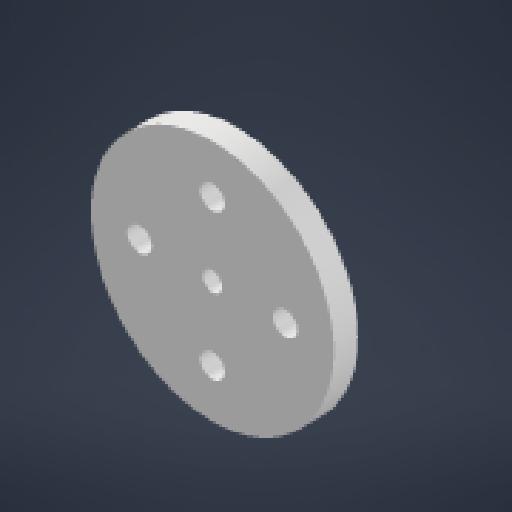
# Autodesk Inventor part: Part25
Saved by Autodesk Inventor 2027.1 (Build 311270010, 270A)
## iProperties
Created: 2026-09-29
Part Number: Part25
Material: Generic
Document SubType Name: Modeling
Designer: daniel
Density: 1 g/cm^3
Appearance: Default
Author: daniel
Autodesk Inventor part; units mm, degrees
ref_plane "YZ Plane" through (0, 0, 0) normal (1, 0, 0) x (0, 1, 0)
ref_plane "XZ Plane" through (0, 0, 0) normal (0, 1, 0) x (-1, 0, 0)
ref_plane "XY Plane" through (0, 0, 0) normal (0, 0, 1) x (1, 0, 0)
sketch "Sketch1" plane through (0, 0, 0) normal (0, 0, 1) x (1, 0, 0)
  circle A0 centre (0, 0) radius 2
  circle A1 centre (0, 0) radius 25
  circle A2 centre (0, 0) radius 3.5
  line L0 (-2, -2.8723) -> (-2, 2.8723)
  line L1 (-2.8723, 2) -> (2.8723, 2)
  line L2 (-2.8723, -2) -> (2.8723, -2)
  line L3 (2, -2.8723) -> (2, 2.8723)
  point P0 (2, -2)
  point P1 (2, 0)
  point P2 (-2, 0)
  point P3 (-2, -2)
  point P4 (2, 2)
  point P5 (-2, 2)
  dimension "d4" = 7
  dimension "d0" = 4
  dimension "d1" = 50
  constraints: 8 end point, 3 coincident, 2 centre point, 2 horizontal, 2 vertical, 10 other
  measures "d0" diameter of A0
  measures "d1" diameter of A1
extrude "Extrusion1" add sketch "Sketch1" along normal blind 5 contours L3 L2 A0 | L3 L1 A2 L2 | A0 L1 L3 | A0 L0 L1 | L1 L0 A2 L3 | L2 L0 A0 | L2 L3 A2 L0 | L2 A2 L3 | L3 A2 L1 | L0 L2 A2 L1 | L1 A2 L0 | L0 A2 L2 | A1
extrude "Extrusion2" add sketch "Sketch1" against normal blind 5 contours L3 L2 A0 | A0 L1 L3 | A0 L0 L1 | L1 L0 A2 L3 | L2 L0 A0 | L2 L3 A2 L0 | L2 A2 L3 | L3 A2 L1 | L1 A2 L0 | L0 A2 L2
sketch "Sketch2" plane through (0, 0, 5) normal (0, 0, 1) x (1, 0, 0)
  circle A0 centre (0, 0) radius 2 projected
  circle A1 centre (0, 0) radius 15
  circle A2 centre (-15, 0) radius 2.5
  circle A3 centre (0, 15) radius 2.5
  circle A4 centre (15, 0) radius 2.5
  circle A5 centre (0, -15) radius 2.5
  dimension "d7" = 30
  dimension "d8" = 5
  dimension "d9" = 5
  dimension "d10" = 5
  dimension "d11" = 5
  constraints: 5 centre point, 4 point on circle, 1 coincident
  measures "d7" diameter of A1
  measures "d8" diameter of A2
  measures "d9" diameter of A3
  measures "d10" diameter of A4
  measures "d11" diameter of A5
extrude "Extrusion3" cut sketch "Sketch2" against normal through all contours A1 A4 | A1 A4 | A3 A1 | A1 A3 | A5 A1 | A1 A5 | A2 A1 | A1 A2
body "Solid1"
